Autodesk Fusion 360 part; units mm, degrees
(part 2 of 2)
  line L91 (21.2817, 6.4213) -> (21.3731, 6.0822)
  line L92 (21.3731, 6.0822) -> (22.0486, 6.2643)
  line L93 (22.0486, 6.2643) -> (22.45, 5.8793)
  line L94 (22.45, 5.8793) -> (21.497, 5.6224)
  line L95 (21.497, 5.6224) -> (21.6223, 5.1575)
  line L96 (21.6223, 5.1575) -> (21.2627, 5.0606)
  line L97 (21.2627, 5.0606) -> (21.1374, 5.5255)
  line L98 (21.1374, 5.5255) -> (19.5423, 5.0955)
  spline S235 degree 2 poles (19.5423, 5.0955) (19.3445, 5.0422) (19.2946, 5.0026) knots 0 0 0 1 1 1
  spline S236 degree 2 poles (19.2946, 5.0026) (19.2446, 4.9629) (19.2261, 4.8987) knots 0 0 0 1 1 1
  spline S237 degree 2 poles (19.2261, 4.8987) (19.2076, 4.8345) (19.2353, 4.7317) knots 0 0 0 1 1 1
  spline S238 degree 2 poles (19.2353, 4.7317) (19.2561, 4.6547) (19.308, 4.5337) knots 0 0 0 1 1 1
  line L99 (19.0191, 3.968) -> (22.8775, 4.536)
  line L100 (22.8775, 4.536) -> (22.9473, 4.0623)
  line L101 (22.9473, 4.0623) -> (21.5629, 3.8585)
  spline S239 degree 2 poles (21.5629, 3.8585) (21.996, 3.5834) (22.0703, 3.0781) knots 0 0 0 1 1 1
  spline S240 degree 2 poles (22.0703, 3.0781) (22.1161, 2.7675) (22.0274, 2.5205) knots 0 0 0 1 1 1
  spline S241 degree 2 poles (22.0274, 2.5205) (21.9387, 2.2735) (21.7374, 2.1431) knots 0 0 0 1 1 1
  spline S242 degree 2 poles (21.7374, 2.1431) (21.5361, 2.0126) (21.1255, 1.9522) knots 0 0 0 1 1 1
  line L102 (21.1255, 1.9522) -> (19.3542, 1.6914)
  line L103 (19.3542, 1.6914) -> (19.2845, 2.1652)
  line L104 (19.2845, 2.1652) -> (21.0558, 2.4259)
  spline S243 degree 2 poles (21.0558, 2.4259) (21.4111, 2.4782) (21.5503, 2.656) knots 0 0 0 1 1 1
  spline S244 degree 2 poles (21.5503, 2.656) (21.6895, 2.8338) (21.6481, 3.1154) knots 0 0 0 1 1 1
  spline S245 degree 2 poles (21.6481, 3.1154) (21.6171, 3.326) (21.4805, 3.4954) knots 0 0 0 1 1 1
  spline S246 degree 2 poles (21.4805, 3.4954) (21.344, 3.6649) (21.1455, 3.7164) knots 0 0 0 1 1 1
  spline S247 degree 2 poles (21.1455, 3.7164) (20.947, 3.7678) (20.618, 3.7194) knots 0 0 0 1 1 1
  line L105 (20.618, 3.7194) -> (19.0889, 3.4943)
  line L106 (19.0889, 3.4943) -> (19.0191, 3.968)
  line L107 (20.2952, -0.9828) -> (20.229, -1.477)
  spline S248 degree 2 poles (20.229, -1.477) (19.7966, -1.3556) (19.5604, -1.0366) knots 0 0 0 1 1 1
  spline S249 degree 2 poles (19.5604, -1.0366) (19.3241, -0.7176) (19.3291, -0.2255) knots 0 0 0 1 1 1
  spline S250 degree 2 poles (19.3291, -0.2255) (19.3353, 0.3943) (19.7207, 0.7536) knots 0 0 0 1 1 1
  spline S251 degree 2 poles (19.7207, 0.7536) (20.1061, 1.1129) (20.7951, 1.1059) knots 0 0 0 1 1 1
  spline S252 degree 2 poles (20.7951, 1.1059) (21.508, 1.0987) (21.898, 0.7277) knots 0 0 0 1 1 1
  spline S253 degree 2 poles (21.898, 0.7277) (22.288, 0.3566) (22.2821, -0.2286) knots 0 0 0 1 1 1
  spline S254 degree 2 poles (22.2821, -0.2286) (22.2764, -0.7953) (21.8871, -1.1505) knots 0 0 0 1 1 1
  spline S255 degree 2 poles (21.8871, -1.1505) (21.4977, -1.5057) (20.7981, -1.4987) knots 0 0 0 1 1 1
  spline S256 degree 2 poles (20.7981, -1.4987) (20.7556, -1.4982) (20.6705, -1.4947) knots 0 0 0 1 1 1
  line L108 (20.6705, -1.4947) -> (20.6917, 0.6121)
  spline S257 degree 2 poles (20.6917, 0.6121) (20.2259, 0.5902) (19.9761, 0.356) knots 0 0 0 1 1 1
  spline S258 degree 2 poles (19.9761, 0.356) (19.7263, 0.1217) (19.7228, -0.2321) knots 0 0 0 1 1 1
  spline S259 degree 2 poles (19.7228, -0.2321) (19.7201, -0.4955) (19.8566, -0.6831) knots 0 0 0 1 1 1
  spline S260 degree 2 poles (19.8566, -0.6831) (19.993, -0.8707) (20.2952, -0.9828) knots 0 0 0 1 1 1
  line L109 (21.0851, 0.5816) -> (21.0692, -0.9959)
  spline S261 degree 2 poles (21.0692, -0.9959) (21.426, -0.9676) (21.6057, -0.8204) knots 0 0 0 1 1 1
  spline S262 degree 2 poles (21.6057, -0.8204) (21.8847, -0.5944) (21.8884, -0.23) knots 0 0 0 1 1 1
  spline S263 degree 2 poles (21.8884, -0.23) (21.8917, 0.0999) (21.6732, 0.3269) knots 0 0 0 1 1 1
  spline S264 degree 2 poles (21.6732, 0.3269) (21.4547, 0.5539) (21.0851, 0.5816) knots 0 0 0 1 1 1
  line L110 (19.1426, -3.6298) -> (22.8872, -4.7198)
  line L111 (22.8872, -4.7198) -> (22.6701, -5.4656)
  line L112 (22.6701, -5.4656) -> (19.7607, -5.5802)
  spline S265 degree 2 poles (19.7607, -5.5802) (19.3547, -5.595) (19.1544, -5.5977) knots 0 0 0 1 1 1
  spline S266 degree 2 poles (19.1544, -5.5977) (19.3401, -5.721) (19.6967, -5.9716) knots 0 0 0 1 1 1
  line L113 (19.6967, -5.9716) -> (22.0411, -7.6266)
  line L114 (22.0411, -7.6266) -> (21.847, -8.2932)
  line L115 (21.847, -8.2932) -> (18.1024, -7.2032)
  line L116 (18.1024, -7.2032) -> (18.2415, -6.7256)
  line L117 (18.2415, -6.7256) -> (21.3756, -7.6379)
  line L118 (21.3756, -7.6379) -> (18.5582, -5.6375)
  line L119 (18.5582, -5.6375) -> (18.6883, -5.1905)
  line L120 (18.6883, -5.1905) -> (22.1913, -5.0353)
  line L121 (22.1913, -5.0353) -> (19.0035, -4.1074)
  line L122 (19.0035, -4.1074) -> (19.1426, -3.6298)
  line L123 (18.9246, -8.4047) -> (18.7313, -8.8535)
  spline S267 degree 2 poles (18.7313, -8.8535) (18.4572, -8.7452) (18.2322, -8.7675) knots 0 0 0 1 1 1
  spline S268 degree 2 poles (18.2322, -8.7675) (18.0072, -8.7899) (17.7791, -8.9692) knots 0 0 0 1 1 1
  spline S269 degree 2 poles (17.7791, -8.9692) (17.5511, -9.1486) (17.3935, -9.4414) knots 0 0 0 1 1 1
  spline S270 degree 2 poles (17.3935, -9.4414) (17.2535, -9.7014) (17.2236, -9.9421) knots 0 0 0 1 1 1
  spline S271 degree 2 poles (17.2236, -9.9421) (17.1936, -10.1828) (17.276, -10.3526) knots 0 0 0 1 1 1
  spline S272 degree 2 poles (17.276, -10.3526) (17.3583, -10.5223) (17.5176, -10.6081) knots 0 0 0 1 1 1
  spline S273 degree 2 poles (17.5176, -10.6081) (17.6792, -10.6951) (17.8503, -10.6663) knots 0 0 0 1 1 1
  spline S274 degree 2 poles (17.8503, -10.6663) (18.0214, -10.6376) (18.2194, -10.4663) knots 0 0 0 1 1 1
  spline S275 degree 2 poles (18.2194, -10.4663) (18.3477, -10.3571) (18.7161, -9.9451) knots 0 0 0 1 1 1
  spline S276 degree 2 poles (18.7161, -9.9451) (19.0844, -9.5331) (19.2873, -9.3976) knots 0 0 0 1 1 1
  spline S277 degree 2 poles (19.2873, -9.3976) (19.5486, -9.2211) (19.8044, -9.2032) knots 0 0 0 1 1 1
  spline S278 degree 2 poles (19.8044, -9.2032) (20.0603, -9.1854) (20.2969, -9.3128) knots 0 0 0 1 1 1
  spline S279 degree 2 poles (20.2969, -9.3128) (20.5569, -9.4528) (20.7034, -9.722) knots 0 0 0 1 1 1
  spline S280 degree 2 poles (20.7034, -9.722) (20.85, -9.9913) (20.8145, -10.3378) knots 0 0 0 1 1 1
  spline S281 degree 2 poles (20.8145, -10.3378) (20.779, -10.6843) (20.5923, -11.031) knots 0 0 0 1 1 1
  spline S282 degree 2 poles (20.5923, -11.031) (20.3868, -11.4127) (20.1068, -11.6382) knots 0 0 0 1 1 1
  spline S283 degree 2 poles (20.1068, -11.6382) (19.8268, -11.8636) (19.5033, -11.8918) knots 0 0 0 1 1 1
  spline S284 degree 2 poles (19.5033, -11.8918) (19.1799, -11.9201) (18.8715, -11.7691) knots 0 0 0 1 1 1
  line L124 (18.8715, -11.7691) -> (19.0733, -11.3158)
  spline S285 degree 2 poles (19.0733, -11.3158) (19.4178, -11.456) (19.6932, -11.3429) knots 0 0 0 1 1 1
  spline S286 degree 2 poles (19.6932, -11.3429) (19.9686, -11.2299) (20.1817, -10.834) knots 0 0 0 1 1 1
  spline S287 degree 2 poles (20.1817, -10.834) (20.4037, -10.4218) (20.3542, -10.1519) knots 0 0 0 1 1 1
  spline S288 degree 2 poles (20.3542, -10.1519) (20.3046, -9.882) (20.0915, -9.7672) knots 0 0 0 1 1 1
  spline S289 degree 2 poles (20.0915, -9.7672) (19.9064, -9.6675) (19.7151, -9.7367) knots 0 0 0 1 1 1
  spline S290 degree 2 poles (19.7151, -9.7367) (19.525, -9.8036) (19.1014, -10.2901) knots 0 0 0 1 1 1
  spline S291 degree 2 poles (19.1014, -10.2901) (18.6778, -10.7765) (18.4731, -10.9322) knots 0 0 0 1 1 1
  spline S292 degree 2 poles (18.4731, -10.9322) (18.1735, -11.1576) (17.8845, -11.1863) knots 0 0 0 1 1 1
  spline S293 degree 2 poles (17.8845, -11.1863) (17.5956, -11.2151) (17.3192, -11.0662) knots 0 0 0 1 1 1
  spline S294 degree 2 poles (17.3192, -11.0662) (17.0452, -10.9187) (16.8873, -10.6312) knots 0 0 0 1 1 1
  spline S295 degree 2 poles (16.8873, -10.6312) (16.7293, -10.3437) (16.7529, -9.9772) knots 0 0 0 1 1 1
  spline S296 degree 2 poles (16.7529, -9.9772) (16.7765, -9.6108) (16.9746, -9.243) knots 0 0 0 1 1 1
  spline S297 degree 2 poles (16.9746, -9.243) (17.2255, -8.7769) (17.531, -8.535) knots 0 0 0 1 1 1
  spline S298 degree 2 poles (17.531, -8.535) (17.8365, -8.2931) (18.2059, -8.2609) knots 0 0 0 1 1 1
  spline S299 degree 2 poles (18.2059, -8.2609) (18.5753, -8.2286) (18.9246, -8.4047) knots 0 0 0 1 1 1
  line L125 (15.066, -12.3544) -> (17.8311, -15.1046)
  line L126 (17.8311, -15.1046) -> (17.2833, -15.6554)
  line L127 (17.2833, -15.6554) -> (14.6745, -14.3626)
  spline S300 degree 2 poles (14.6745, -14.3626) (14.3109, -14.1811) (14.1339, -14.0875) knots 0 0 0 1 1 1
  spline S301 degree 2 poles (14.1339, -14.0875) (14.2379, -14.2848) (14.4308, -14.6755) knots 0 0 0 1 1 1
  line L128 (14.4308, -14.6755) -> (15.6962, -17.2511)
  line L129 (15.6962, -17.2511) -> (15.2066, -17.7434)
  line L130 (15.2066, -17.7434) -> (12.4414, -14.9932)
  line L131 (12.4414, -14.9932) -> (12.7922, -14.6405)
  line L132 (12.7922, -14.6405) -> (15.1066, -16.9423)
  line L133 (15.1066, -16.9423) -> (13.5914, -13.8369)
  line L134 (13.5914, -13.8369) -> (13.9197, -13.5068)
  line L135 (13.9197, -13.5068) -> (17.0691, -15.0484)
  line L136 (17.0691, -15.0484) -> (14.7152, -12.7071)
  line L137 (14.7152, -12.7071) -> (15.066, -12.3544)
  line L138 (11.1944, -14.5207) -> (11.4925, -14.8614)
  spline S302 degree 2 poles (11.4925, -14.8614) (11.3389, -14.9151) (11.2424, -14.9813) knots 0 0 0 1 1 1
  spline S303 degree 2 poles (11.2424, -14.9813) (11.1107, -15.0715) (11.0618, -15.1695) knots 0 0 0 1 1 1
  spline S304 degree 2 poles (11.0618, -15.1695) (11.0129, -15.2676) (11.0166, -15.3811) knots 0 0 0 1 1 1
  spline S305 degree 2 poles (11.0166, -15.3811) (11.0199, -15.466) (11.0974, -15.7579) knots 0 0 0 1 1 1
  spline S306 degree 2 poles (11.0974, -15.7579) (11.109, -15.7983) (11.1285, -15.8785) knots 0 0 0 1 1 1
  line L139 (11.1285, -15.8785) -> (13.6131, -17.6072)
  line L140 (13.6131, -17.6072) -> (13.1874, -17.899)
  line L141 (13.1874, -17.899) -> (11.7775, -16.8818)
  spline S307 degree 2 poles (11.7775, -16.8818) (11.5071, -16.6898) (11.2385, -16.4578) knots 0 0 0 1 1 1
  spline S308 degree 2 poles (11.2385, -16.4578) (11.357, -16.7766) (11.4401, -17.1002) knots 0 0 0 1 1 1
  line L142 (11.4401, -17.1002) -> (11.873, -18.7999)
  line L143 (11.873, -18.7999) -> (11.478, -19.0706)
  line L144 (11.478, -19.0706) -> (10.7402, -16.0931)
  spline S309 degree 2 poles (10.7402, -16.0931) (10.6196, -15.6113) (10.5993, -15.4123) knots 0 0 0 1 1 1
  spline S310 degree 2 poles (10.5993, -15.4123) (10.5708, -15.1449) (10.6444, -14.9605) knots 0 0 0 1 1 1
  spline S311 degree 2 poles (10.6444, -14.9605) (10.718, -14.7762) (10.9068, -14.6469) knots 0 0 0 1 1 1
  spline S312 degree 2 poles (10.9068, -14.6469) (11.0209, -14.5687) (11.1944, -14.5207) knots 0 0 0 1 1 1
  line L145 (10.0619, -17.5995) -> (9.6708, -17.8766)
  spline S313 degree 2 poles (9.6708, -17.8766) (9.5086, -17.6394) (9.2779, -17.5845) knots 0 0 0 1 1 1
  spline S314 degree 2 poles (9.2779, -17.5845) (9.0473, -17.5296) (8.7542, -17.675) knots 0 0 0 1 1 1
  spline S315 degree 2 poles (8.7542, -17.675) (8.4586, -17.8216) (8.3753, -18.0128) knots 0 0 0 1 1 1
  spline S316 degree 2 poles (8.3753, -18.0128) (8.292, -18.2041) (8.3724, -18.3662) knots 0 0 0 1 1 1
  spline S317 degree 2 poles (8.3724, -18.3662) (8.4445, -18.5116) (8.6122, -18.5323) knots 0 0 0 1 1 1
  spline S318 degree 2 poles (8.6122, -18.5323) (8.7287, -18.5458) (9.1228, -18.4602) knots 0 0 0 1 1 1
  spline S319 degree 2 poles (9.1228, -18.4602) (9.6538, -18.3453) (9.8793, -18.3419) knots 0 0 0 1 1 1
  spline S320 degree 2 poles (9.8793, -18.3419) (10.1047, -18.3385) (10.2751, -18.4455) knots 0 0 0 1 1 1
  spline S321 degree 2 poles (10.2751, -18.4455) (10.4455, -18.5525) (10.5377, -18.7384) knots 0 0 0 1 1 1
  spline S322 degree 2 poles (10.5377, -18.7384) (10.6216, -18.9077) (10.6157, -19.0903) knots 0 0 0 1 1 1
  spline S323 degree 2 poles (10.6157, -19.0903) (10.6097, -19.2729) (10.5235, -19.4344) knots 0 0 0 1 1 1
  spline S324 degree 2 poles (10.5235, -19.4344) (10.4601, -19.5579) (10.3127, -19.6948) knots 0 0 0 1 1 1
  spline S325 degree 2 poles (10.3127, -19.6948) (10.1653, -19.8318) (9.9675, -19.9299) knots 0 0 0 1 1 1
  spline S326 degree 2 poles (9.9675, -19.9299) (9.6696, -20.0776) (9.4018, -20.1035) knots 0 0 0 1 1 1
  spline S327 degree 2 poles (9.4018, -20.1035) (9.1341, -20.1294) (8.9541, -20.0361) knots 0 0 0 1 1 1
  spline S328 degree 2 poles (8.9541, -20.0361) (8.7742, -19.9427) (8.6119, -19.7173) knots 0 0 0 1 1 1
  line L146 (8.6119, -19.7173) -> (9.003, -19.4521)
  spline S329 degree 2 poles (9.003, -19.4521) (9.1285, -19.6333) (9.3199, -19.675) knots 0 0 0 1 1 1
  spline S330 degree 2 poles (9.3199, -19.675) (9.5113, -19.7166) (9.7616, -19.5925) knots 0 0 0 1 1 1
  spline S331 degree 2 poles (9.7616, -19.5925) (10.0571, -19.446) (10.135, -19.2856) knots 0 0 0 1 1 1
  spline S332 degree 2 poles (10.135, -19.2856) (10.2128, -19.1252) (10.1478, -18.9942) knots 0 0 0 1 1 1
  spline S333 degree 2 poles (10.1478, -18.9942) (10.1064, -18.9107) (10.0209, -18.87) knots 0 0 0 1 1 1
  spline S334 degree 2 poles (10.0209, -18.87) (9.9342, -18.8269) (9.7997, -18.8372) knots 0 0 0 1 1 1
  spline S335 degree 2 poles (9.7997, -18.8372) (9.7236, -18.8453) (9.3664, -18.9155) knots 0 0 0 1 1 1
  spline S336 degree 2 poles (9.3664, -18.9155) (8.8509, -19.0197) (8.6326, -19.0315) knots 0 0 0 1 1 1
  spline S337 degree 2 poles (8.6326, -19.0315) (8.4142, -19.0433) (8.2385, -18.9463) knots 0 0 0 1 1 1
  spline S338 degree 2 poles (8.2385, -18.9463) (8.0627, -18.8494) (7.9539, -18.6301) knots 0 0 0 1 1 1
  spline S339 degree 2 poles (7.9539, -18.6301) (7.8476, -18.4156) (7.8787, -18.1641) knots 0 0 0 1 1 1
  spline S340 degree 2 poles (7.8787, -18.1641) (7.9099, -17.9126) (8.0944, -17.6919) knots 0 0 0 1 1 1
  spline S341 degree 2 poles (8.0944, -17.6919) (8.2789, -17.4712) (8.5768, -17.3234) knots 0 0 0 1 1 1
  spline S342 degree 2 poles (8.5768, -17.3234) (9.0702, -17.0788) (9.4304, -17.1555) knots 0 0 0 1 1 1
  spline S343 degree 2 poles (9.4304, -17.1555) (9.7907, -17.2322) (10.0619, -17.5995) knots 0 0 0 1 1 1
  line L147 (6.2103, -18.8357) -> (5.9999, -18.4623)
  spline S344 degree 2 poles (5.9999, -18.4623) (6.1751, -18.3528) (6.3249, -18.2979) knots 0 0 0 1 1 1
  spline S345 degree 2 poles (6.3249, -18.2979) (6.5697, -18.2082) (6.733, -18.2363) knots 0 0 0 1 1 1
  spline S346 degree 2 poles (6.733, -18.2363) (6.8963, -18.2643) (6.9974, -18.3703) knots 0 0 0 1 1 1
  spline S347 degree 2 poles (6.9974, -18.3703) (7.0986, -18.4763) (7.2468, -18.881) knots 0 0 0 1 1 1
  line L148 (7.2468, -18.881) -> (7.806, -20.4072)
  line L149 (7.806, -20.4072) -> (8.1357, -20.2865)
  line L150 (8.1357, -20.2865) -> (8.2638, -20.6362)
  line L151 (8.2638, -20.6362) -> (7.9341, -20.757)
  line L152 (7.9341, -20.757) -> (8.1747, -21.4139)
  line L153 (8.1747, -21.4139) -> (7.8264, -21.8475)
  line L154 (7.8264, -21.8475) -> (7.4869, -20.9208)
  line L155 (7.4869, -20.9208) -> (7.0348, -21.0864)
  line L156 (7.0348, -21.0864) -> (6.9067, -20.7367)
  line L157 (6.9067, -20.7367) -> (7.3588, -20.571)
  line L158 (7.3588, -20.571) -> (6.7905, -19.0198)
  spline S348 degree 2 poles (6.7905, -19.0198) (6.7201, -18.8275) (6.6762, -18.7812) knots 0 0 0 1 1 1
  spline S349 degree 2 poles (6.6762, -18.7812) (6.6324, -18.7349) (6.5668, -18.7221) knots 0 0 0 1 1 1
  spline S350 degree 2 poles (6.5668, -18.7221) (6.5012, -18.7094) (6.4012, -18.746) knots 0 0 0 1 1 1
  spline S351 degree 2 poles (6.4012, -18.746) (6.3263, -18.7734) (6.2103, -18.8357) knots 0 0 0 1 1 1
  line L159 (6.5393, -21.7845) -> (6.692, -22.3136)
  line L160 (6.692, -22.3136) -> (6.2319, -22.4464)
  line L161 (6.2319, -22.4464) -> (6.0792, -21.9173)
  line L162 (6.0792, -21.9173) -> (6.5393, -21.7845)
  line L163 (5.6108, -18.5665) -> (6.394, -21.281)
  line L164 (6.394, -21.281) -> (5.9339, -21.4137)
  line L165 (5.9339, -21.4137) -> (5.1507, -18.6993)
  line L166 (5.1507, -18.6993) -> (5.6108, -18.5665)
  line L167 (2.4912, -18.1527) -> (2.7274, -19.5158)
  spline S352 degree 2 poles (2.7274, -19.5158) (2.8107, -19.342) (2.9908, -19.2055) knots 0 0 0 1 1 1
  spline S353 degree 2 poles (2.9908, -19.2055) (3.171, -19.069) (3.3938, -19.0304) knots 0 0 0 1 1 1
  spline S354 degree 2 poles (3.3938, -19.0304) (3.8893, -18.9445) (4.3156, -19.2783) knots 0 0 0 1 1 1
  spline S355 degree 2 poles (4.3156, -19.2783) (4.742, -19.6121) (4.8615, -20.3015) knots 0 0 0 1 1 1
  spline S356 degree 2 poles (4.8615, -20.3015) (4.9342, -20.7209) (4.8464, -21.079) knots 0 0 0 1 1 1
  spline S357 degree 2 poles (4.8464, -21.079) (4.7586, -21.4371) (4.5118, -21.6567) knots 0 0 0 1 1 1
  spline S358 degree 2 poles (4.5118, -21.6567) (4.265, -21.8763) (3.9348, -21.9336) knots 0 0 0 1 1 1
  spline S359 degree 2 poles (3.9348, -21.9336) (3.4184, -22.0231) (3.0468, -21.6393) knots 0 0 0 1 1 1
  line L168 (3.0468, -21.6393) -> (3.1113, -22.0115)
  line L169 (3.1113, -22.0115) -> (2.6866, -22.0851)
  line L170 (2.6866, -22.0851) -> (2.0193, -18.2345)
  line L171 (2.0193, -18.2345) -> (2.4912, -18.1527)
  spline S360 degree 2 poles (4.3734, -20.3672) (4.2803, -19.8298) (4.0083, -19.6002) knots 0 0 0 1 1 1
  spline S361 degree 2 poles (4.0083, -19.6002) (3.7363, -19.3706) (3.4218, -19.4251) knots 0 0 0 1 1 1
  spline S362 degree 2 poles (3.4218, -19.4251) (3.1203, -19.4774) (2.947, -19.7706) knots 0 0 0 1 1 1
  spline S363 degree 2 poles (2.947, -19.7706) (2.7738, -20.0639) (2.8642, -20.5855) knots 0 0 0 1 1 1
  spline S364 degree 2 poles (2.8642, -20.5855) (2.9605, -21.1412) (3.2384, -21.3819) knots 0 0 0 1 1 1
  spline S365 degree 2 poles (3.2384, -21.3819) (3.5164, -21.6227) (3.8257, -21.5691) knots 0 0 0 1 1 1
  spline S366 degree 2 poles (3.8257, -21.5691) (4.1324, -21.5159) (4.3008, -21.2181) knots 0 0 0 1 1 1
  spline S367 degree 2 poles (4.3008, -21.2181) (4.4692, -20.9203) (4.3734, -20.3672) knots 0 0 0 1 1 1
  line L172 (-0.3977, -19.4026) -> (-0.3913, -19.8176)
  spline S368 degree 2 poles (-0.3913, -19.8176) (-0.0688, -19.3337) (0.4978, -19.325) knots 0 0 0 1 1 1
  spline S369 degree 2 poles (0.4978, -19.325) (0.7478, -19.3212) (0.966, -19.4136) knots 0 0 0 1 1 1
  spline S370 degree 2 poles (0.966, -19.4136) (1.1843, -19.506) (1.2916, -19.6494) knots 0 0 0 1 1 1
  spline S371 degree 2 poles (1.2916, -19.6494) (1.3989, -19.7927) (1.4447, -20.0022) knots 0 0 0 1 1 1
  spline S372 degree 2 poles (1.4447, -20.0022) (1.4761, -20.1428) (1.4808, -20.4487) knots 0 0 0 1 1 1
  line L173 (1.4808, -20.4487) -> (1.5077, -22.1989)
  line L174 (1.5077, -22.1989) -> (1.0289, -22.2063)
  line L175 (1.0289, -22.2063) -> (1.0048, -20.6396)
  spline S373 degree 2 poles (1.0048, -20.6396) (0.9991, -20.2645) (0.9678, -20.1346) knots 0 0 0 1 1 1
  spline S374 degree 2 poles (0.9678, -20.1346) (0.9197, -19.9464) (0.7717, -19.841) knots 0 0 0 1 1 1
  spline S375 degree 2 poles (0.7717, -19.841) (0.6238, -19.7355) (0.4083, -19.7388) knots 0 0 0 1 1 1
  spline S376 degree 2 poles (0.4083, -19.7388) (0.1929, -19.7421) (0.0057, -19.8554) knots 0 0 0 1 1 1
  spline S377 degree 2 poles (0.0057, -19.8554) (-0.1815, -19.9687) (-0.257, -20.1601) knots 0 0 0 1 1 1
  spline S378 degree 2 poles (-0.257, -20.1601) (-0.3326, -20.3515) (-0.327, -20.7132) knots 0 0 0 1 1 1
  line L176 (-0.327, -20.7132) -> (-0.3037, -22.2268)
  line L177 (-0.3037, -22.2268) -> (-0.7825, -22.2341)
  line L178 (-0.7825, -22.2341) -> (-0.8259, -19.4092)
  line L179 (-0.8259, -19.4092) -> (-0.3977, -19.4026)
  line L180 (-3.6213, -19.9937) -> (-4.1026, -19.8636)
  spline S379 degree 2 poles (-4.1026, -19.8636) (-3.9259, -19.4507) (-3.5788, -19.2581) knots 0 0 0 1 1 1
  spline S380 degree 2 poles (-3.5788, -19.2581) (-3.2317, -19.0655) (-2.7445, -19.1346) knots 0 0 0 1 1 1
  spline S381 degree 2 poles (-2.7445, -19.1346) (-2.1308, -19.2216) (-1.8248, -19.6506) knots 0 0 0 1 1 1
  spline S382 degree 2 poles (-1.8248, -19.6506) (-1.5189, -20.0795) (-1.6156, -20.7617) knots 0 0 0 1 1 1
  spline S383 degree 2 poles (-1.6156, -20.7617) (-1.7157, -21.4676) (-2.1345, -21.8059) knots 0 0 0 1 1 1
  spline S384 degree 2 poles (-2.1345, -21.8059) (-2.5533, -22.1442) (-3.1327, -22.062) knots 0 0 0 1 1 1
  spline S385 degree 2 poles (-3.1327, -22.062) (-3.6938, -21.9824) (-3.9952, -21.5501) knots 0 0 0 1 1 1
  spline S386 degree 2 poles (-3.9952, -21.5501) (-4.2966, -21.1177) (-4.1984, -20.425) knots 0 0 0 1 1 1
  spline S387 degree 2 poles (-4.1984, -20.425) (-4.1924, -20.3829) (-4.1778, -20.299) knots 0 0 0 1 1 1
  line L181 (-4.1778, -20.299) -> (-2.0917, -20.5948)
  spline S388 degree 2 poles (-2.0917, -20.5948) (-2.0527, -20.1301) (-2.2524, -19.8519) knots 0 0 0 1 1 1
  spline S389 degree 2 poles (-2.2524, -19.8519) (-2.4521, -19.5737) (-2.8024, -19.524) knots 0 0 0 1 1 1
  spline S390 degree 2 poles (-2.8024, -19.524) (-3.0631, -19.4871) (-3.2669, -19.5979) knots 0 0 0 1 1 1
  spline S391 degree 2 poles (-3.2669, -19.5979) (-3.4707, -19.7087) (-3.6213, -19.9937) knots 0 0 0 1 1 1
  line L182 (-2.1734, -20.9809) -> (-3.7353, -20.7594)
  spline S392 degree 2 poles (-3.7353, -20.7594) (-3.7537, -21.1168) (-3.6313, -21.3142) knots 0 0 0 1 1 1
  spline S393 degree 2 poles (-3.6313, -21.3142) (-3.4436, -21.6203) (-3.0827, -21.6714) knots 0 0 0 1 1 1
  spline S394 degree 2 poles (-3.0827, -21.6714) (-2.7561, -21.7178) (-2.5026, -21.5307) knots 0 0 0 1 1 1
  spline S395 degree 2 poles (-2.5026, -21.5307) (-2.249, -21.3436) (-2.1734, -20.9809) knots 0 0 0 1 1 1
  spline S396 degree 2 poles (-6.3827, -19.8486) (-6.6703, -20.5788) (-7.2147, -20.7704) knots 0 0 0 1 1 1
  spline S397 degree 2 poles (-7.2147, -20.7704) (-7.6688, -20.9289) (-8.1564, -20.7369) knots 0 0 0 1 1 1
  spline S398 degree 2 poles (-8.1564, -20.7369) (-8.6985, -20.5234) (-8.9027, -20.0327) knots 0 0 0 1 1 1
  spline S399 degree 2 poles (-8.9027, -20.0327) (-9.1069, -19.542) (-8.8603, -18.9158) knots 0 0 0 1 1 1
  spline S400 degree 2 poles (-8.8603, -18.9158) (-8.6604, -18.4083) (-8.3937, -18.1774) knots 0 0 0 1 1 1
  spline S401 degree 2 poles (-8.3937, -18.1774) (-8.1269, -17.9466) (-7.7727, -17.9002) knots 0 0 0 1 1 1
  spline S402 degree 2 poles (-7.7727, -17.9002) (-7.4185, -17.8538) (-7.0744, -17.9893) knots 0 0 0 1 1 1
  spline S403 degree 2 poles (-7.0744, -17.9893) (-6.5224, -18.2067) (-6.3215, -18.6947) knots 0 0 0 1 1 1
  spline S404 degree 2 poles (-6.3215, -18.6947) (-6.1205, -19.1827) (-6.3827, -19.8486) knots 0 0 0 1 1 1
  spline S405 degree 2 poles (-6.8407, -19.6682) (-6.6418, -19.1633) (-6.7632, -18.8253) knots 0 0 0 1 1 1
  spline S406 degree 2 poles (-6.7632, -18.8253) (-6.8845, -18.4873) (-7.2187, -18.3557) knots 0 0 0 1 1 1
  spline S407 degree 2 poles (-7.2187, -18.3557) (-7.5504, -18.2251) (-7.8701, -18.3908) knots 0 0 0 1 1 1
  spline S408 degree 2 poles (-7.8701, -18.3908) (-8.1898, -18.5565) (-8.3936, -19.0738) knots 0 0 0 1 1 1
  spline S409 degree 2 poles (-8.3936, -19.0738) (-8.5856, -19.5615) (-8.463, -19.8999) knots 0 0 0 1 1 1
  spline S410 degree 2 poles (-8.463, -19.8999) (-8.3404, -20.2384) (-8.0112, -20.3681) knots 0 0 0 1 1 1
  spline S411 degree 2 poles (-8.0112, -20.3681) (-7.677, -20.4997) (-7.3583, -20.3364) knots 0 0 0 1 1 1
  spline S412 degree 2 poles (-7.3583, -20.3364) (-7.0395, -20.1732) (-6.8407, -19.6682) knots 0 0 0 1 1 1
  line L183 (-8.9179, -17.2264) -> (-10.0878, -19.3823)
  line L184 (-10.0878, -19.3823) -> (-9.716, -19.584)
  line L185 (-9.716, -19.584) -> (-9.8936, -19.9114)
  line L186 (-9.8936, -19.9114) -> (-10.2654, -19.7096)
  line L187 (-10.2654, -19.7096) -> (-10.4088, -19.9738)
  spline S413 degree 2 poles (-10.4088, -19.9738) (-10.5445, -20.224) (-10.6549, -20.3215) knots 0 0 0 1 1 1
  spline S414 degree 2 poles (-10.6549, -20.3215) (-10.8045, -20.4522) (-11.0129, -20.4708) knots 0 0 0 1 1 1
  spline S415 degree 2 poles (-11.0129, -20.4708) (-11.2212, -20.4894) (-11.4972, -20.3397) knots 0 0 0 1 1 1
  spline S416 degree 2 poles (-11.4972, -20.3397) (-11.6749, -20.2433) (-11.8671, -20.0844) knots 0 0 0 1 1 1
  line L188 (-11.8671, -20.0844) -> (-11.6048, -19.7516)
  spline S417 degree 2 poles (-11.6048, -19.7516) (-11.4865, -19.846) (-11.3696, -19.9095) knots 0 0 0 1 1 1
  spline S418 degree 2 poles (-11.3696, -19.9095) (-11.1779, -20.0135) (-11.054, -19.9748) knots 0 0 0 1 1 1
  spline S419 degree 2 poles (-11.054, -19.9748) (-10.9301, -19.9361) (-10.8083, -19.7117) knots 0 0 0 1 1 1
  line L189 (-10.8083, -19.7117) -> (-10.6839, -19.4825)
  line L190 (-10.6839, -19.4825) -> (-11.168, -19.2199)
  line L191 (-11.168, -19.2199) -> (-10.9903, -18.8925)
  line L192 (-10.9903, -18.8925) -> (-10.5063, -19.1552)
  line L193 (-10.5063, -19.1552) -> (-9.3365, -16.9993)
  line L194 (-9.3365, -16.9993) -> (-8.9179, -17.2264)
  line L195 (-11.5378, -15.5911) -> (-13.899, -18.695)
  line L196 (-13.899, -18.695) -> (-14.2801, -18.4051)
  line L197 (-14.2801, -18.4051) -> (-11.9189, -15.3011)
  line L198 (-11.9189, -15.3011) -> (-11.5378, -15.5911)
  line L199 (-14.5469, -14.1862) -> (-14.8636, -13.801)
  spline S420 degree 2 poles (-14.8636, -13.801) (-14.4801, -13.5672) (-14.0856, -13.6116) knots 0 0 0 1 1 1
  spline S421 degree 2 poles (-14.0856, -13.6116) (-13.6912, -13.656) (-13.3344, -13.995) knots 0 0 0 1 1 1
  spline S422 degree 2 poles (-13.3344, -13.995) (-12.8849, -14.4219) (-12.8845, -14.9487) knots 0 0 0 1 1 1
  spline S423 degree 2 poles (-12.8845, -14.9487) (-12.8841, -15.4756) (-13.3586, -15.9752) knots 0 0 0 1 1 1
  spline S424 degree 2 poles (-13.3586, -15.9752) (-13.8496, -16.4921) (-14.387, -16.5248) knots 0 0 0 1 1 1
  spline S425 degree 2 poles (-14.387, -16.5248) (-14.9243, -16.5575) (-15.3487, -16.1544) knots 0 0 0 1 1 1
  spline S426 degree 2 poles (-15.3487, -16.1544) (-15.7595, -15.7642) (-15.7543, -15.2372) knots 0 0 0 1 1 1
  spline S427 degree 2 poles (-15.7543, -15.2372) (-15.749, -14.7101) (-15.2672, -14.2028) knots 0 0 0 1 1 1
  spline S428 degree 2 poles (-15.2672, -14.2028) (-15.2379, -14.172) (-15.1773, -14.1121) knots 0 0 0 1 1 1
  line L200 (-15.1773, -14.1121) -> (-13.6496, -15.5631)
  spline S429 degree 2 poles (-13.6496, -15.5631) (-13.3483, -15.2072) (-13.3496, -14.8647) knots 0 0 0 1 1 1
  spline S430 degree 2 poles (-13.3496, -14.8647) (-13.3509, -14.5223) (-13.6074, -14.2786) knots 0 0 0 1 1 1
  spline S431 degree 2 poles (-13.6074, -14.2786) (-13.7984, -14.0973) (-14.0287, -14.0693) knots 0 0 0 1 1 1
  spline S432 degree 2 poles (-14.0287, -14.0693) (-14.259, -14.0414) (-14.5469, -14.1862) knots 0 0 0 1 1 1
  line L201 (-13.9401, -15.8302) -> (-15.0839, -14.7438)
  spline S433 degree 2 poles (-15.0839, -14.7438) (-15.3063, -15.0243) (-15.321, -15.2561) knots 0 0 0 1 1 1
  spline S434 degree 2 poles (-15.321, -15.2561) (-15.3456, -15.6143) (-15.0814, -15.8653) knots 0 0 0 1 1 1
  spline S435 degree 2 poles (-15.0814, -15.8653) (-14.8422, -16.0924) (-14.5271, -16.0871) knots 0 0 0 1 1 1
  spline S436 degree 2 poles (-14.5271, -16.0871) (-14.2121, -16.0819) (-13.9401, -15.8302) knots 0 0 0 1 1 1
  line L202 (-15.8662, -11.1763) -> (-15.6239, -11.5486)
  line L203 (-15.6239, -11.5486) -> (-18.8928, -13.6757)
  line L204 (-18.8928, -13.6757) -> (-19.154, -13.2743)
  line L205 (-19.154, -13.2743) -> (-17.9878, -12.5155)
  spline S437 degree 2 poles (-17.9878, -12.5155) (-18.4721, -12.4688) (-18.7289, -12.0741) knots 0 0 0 1 1 1
  spline S438 degree 2 poles (-18.7289, -12.0741) (-18.8711, -11.8556) (-18.91, -11.6032) knots 0 0 0 1 1 1
  spline S439 degree 2 poles (-18.91, -11.6032) (-18.9488, -11.3507) (-18.8714, -11.121) knots 0 0 0 1 1 1
  spline S440 degree 2 poles (-18.8714, -11.121) (-18.7939, -10.8913) (-18.6151, -10.6734) knots 0 0 0 1 1 1
  spline S441 degree 2 poles (-18.6151, -10.6734) (-18.4364, -10.4555) (-18.1799, -10.2886) knots 0 0 0 1 1 1
  spline S442 degree 2 poles (-18.1799, -10.2886) (-17.5712, -9.8925) (-17.0431, -9.9774) knots 0 0 0 1 1 1
  spline S443 degree 2 poles (-17.0431, -9.9774) (-16.515, -10.0622) (-16.2407, -10.4836) knots 0 0 0 1 1 1
  spline S444 degree 2 poles (-16.2407, -10.4836) (-15.968, -10.9029) (-16.1628, -11.3692) knots 0 0 0 1 1 1
  line L206 (-16.1628, -11.3692) -> (-15.8662, -11.1763)
  spline S445 degree 2 poles (-17.0652, -11.9628) (-16.6393, -11.6856) (-16.5252, -11.4464) knots 0 0 0 1 1 1
  spline S446 degree 2 poles (-16.5252, -11.4464) (-16.3386, -11.0552) (-16.549, -10.7318) knots 0 0 0 1 1 1
  spline S447 degree 2 poles (-16.549, -10.7318) (-16.7202, -10.4687) (-17.0735, -10.4257) knots 0 0 0 1 1 1
  spline S448 degree 2 poles (-17.0735, -10.4257) (-17.4269, -10.3826) (-17.8795, -10.6772) knots 0 0 0 1 1 1
  spline S449 degree 2 poles (-17.8795, -10.6772) (-18.3433, -10.979) (-18.4444, -11.3066) knots 0 0 0 1 1 1
  spline S450 degree 2 poles (-18.4444, -11.3066) (-18.5454, -11.6342) (-18.3757, -11.895) knots 0 0 0 1 1 1
  spline S451 degree 2 poles (-18.3757, -11.895) (-18.2045, -12.1582) (-17.8511, -12.2012) knots 0 0 0 1 1 1
  spline S452 degree 2 poles (-17.8511, -12.2012) (-17.4978, -12.2442) (-17.0652, -11.9628) knots 0 0 0 1 1 1
  spline S453 degree 2 poles (-18.4484, -9.714) (-19.1648, -10.0344) (-19.6878, -9.7904) knots 0 0 0 1 1 1
  spline S454 degree 2 poles (-19.6878, -9.7904) (-20.1232, -9.5859) (-20.3371, -9.1075) knots 0 0 0 1 1 1
  spline S455 degree 2 poles (-20.3371, -9.1075) (-20.575, -8.5757) (-20.3776, -8.0823) knots 0 0 0 1 1 1
  spline S456 degree 2 poles (-20.3776, -8.0823) (-20.1801, -7.5888) (-19.5657, -7.314) knots 0 0 0 1 1 1
  spline S457 degree 2 poles (-19.5657, -7.314) (-19.0679, -7.0913) (-18.7157, -7.113) knots 0 0 0 1 1 1
  spline S458 degree 2 poles (-18.7157, -7.113) (-18.3636, -7.1347) (-18.0781, -7.3494) knots 0 0 0 1 1 1
  spline S459 degree 2 poles (-18.0781, -7.3494) (-17.7926, -7.5642) (-17.6416, -7.9017) knots 0 0 0 1 1 1
  spline S460 degree 2 poles (-17.6416, -7.9017) (-17.3994, -8.4433) (-17.5973, -8.9325) knots 0 0 0 1 1 1
  spline S461 degree 2 poles (-17.5973, -8.9325) (-17.7952, -9.4218) (-18.4484, -9.714) knots 0 0 0 1 1 1
  spline S462 degree 2 poles (-18.6494, -9.2647) (-18.154, -9.0431) (-18.0042, -8.7167) knots 0 0 0 1 1 1
  spline S463 degree 2 poles (-18.0042, -8.7167) (-17.8544, -8.3903) (-18.001, -8.0625) knots 0 0 0 1 1 1
  spline S464 degree 2 poles (-18.001, -8.0625) (-18.1466, -7.7371) (-18.491, -7.6318) knots 0 0 0 1 1 1
  spline S465 degree 2 poles (-18.491, -7.6318) (-18.8353, -7.5264) (-19.3429, -7.7535) knots 0 0 0 1 1 1
  spline S466 degree 2 poles (-19.3429, -7.7535) (-19.8213, -7.9675) (-19.9705, -8.2951) knots 0 0 0 1 1 1
  spline S467 degree 2 poles (-19.9705, -8.2951) (-20.1198, -8.6227) (-19.9753, -8.9456) knots 0 0 0 1 1 1
  spline S468 degree 2 poles (-19.9753, -8.9456) (-19.8287, -9.2735) (-19.4867, -9.3799) knots 0 0 0 1 1 1
  spline S469 degree 2 poles (-19.4867, -9.3799) (-19.1448, -9.4863) (-18.6494, -9.2647) knots 0 0 0 1 1 1
  spline S470 degree 2 poles (-19.2364, -4.4954) (-18.9486, -4.6931) (-18.7944, -4.9063) knots 0 0 0 1 1 1
  spline S471 degree 2 poles (-18.7944, -4.9063) (-18.6403, -5.1195) (-18.5666, -5.3917) knots 0 0 0 1 1 1
  spline S472 degree 2 poles (-18.5666, -5.3917) (-18.4449, -5.8411) (-18.5991, -6.1419) knots 0 0 0 1 1 1
  spline S473 degree 2 poles (-18.5991, -6.1419) (-18.7533, -6.4427) (-19.0949, -6.5351) knots 0 0 0 1 1 1
  spline S474 degree 2 poles (-19.0949, -6.5351) (-19.2951, -6.5894) (-19.4855, -6.5431) knots 0 0 0 1 1 1
  spline S475 degree 2 poles (-19.4855, -6.5431) (-19.6758, -6.4967) (-19.8159, -6.3762) knots 0 0 0 1 1 1
  spline S476 degree 2 poles (-19.8159, -6.3762) (-19.956, -6.2557) (-20.0574, -6.0847) knots 0 0 0 1 1 1
  spline S477 degree 2 poles (-20.0574, -6.0847) (-20.1302, -5.9583) (-20.238, -5.6926) knots 0 0 0 1 1 1
  spline S478 degree 2 poles (-20.238, -5.6926) (-20.4563, -5.1509) (-20.6203, -4.9114) knots 0 0 0 1 1 1
  spline S479 degree 2 poles (-20.6203, -4.9114) (-20.716, -4.9346) (-20.7417, -4.9415) knots 0 0 0 1 1 1
  spline S480 degree 2 poles (-20.7417, -4.9415) (-21.0242, -5.018) (-21.1043, -5.1802) knots 0 0 0 1 1 1
  spline S481 degree 2 poles (-21.1043, -5.1802) (-21.213, -5.3998) (-21.1184, -5.749) knots 0 0 0 1 1 1
  spline S482 degree 2 poles (-21.1184, -5.749) (-21.0301, -6.0752) (-20.8738, -6.1996) knots 0 0 0 1 1 1
  spline S483 degree 2 poles (-20.8738, -6.1996) (-20.7175, -6.324) (-20.4071, -6.3199) knots 0 0 0 1 1 1
  line L207 (-20.4071, -6.3199) -> (-20.3464, -6.7885)
  spline S484 degree 2 poles (-20.3464, -6.7885) (-20.6533, -6.8055) (-20.87, -6.7126) knots 0 0 0 1 1 1
  spline S485 degree 2 poles (-20.87, -6.7126) (-21.0867, -6.6196) (-21.2553, -6.3786) knots 0 0 0 1 1 1
  spline S486 degree 2 poles (-21.2553, -6.3786) (-21.4239, -6.1377) (-21.5191, -5.7859) knots 0 0 0 1 1 1
  spline S487 degree 2 poles (-21.5191, -5.7859) (-21.6136, -5.4366) (-21.5906, -5.1961) knots 0 0 0 1 1 1
  spline S488 degree 2 poles (-21.5906, -5.1961) (-21.5675, -4.9556) (-21.4707, -4.8192) knots 0 0 0 1 1 1
  spline S489 degree 2 poles (-21.4707, -4.8192) (-21.374, -4.6827) (-21.1951, -4.5902) knots 0 0 0 1 1 1
  spline S490 degree 2 poles (-21.1951, -4.5902) (-21.0833, -4.5351) (-20.7751, -4.4517) knots 0 0 0 1 1 1
  line L208 (-20.7751, -4.4517) -> (-20.1588, -4.2849)
  spline S491 degree 2 poles (-20.1588, -4.2849) (-19.5143, -4.1104) (-19.3515, -4.0346) knots 0 0 0 1 1 1
  spline S492 degree 2 poles (-19.3515, -4.0346) (-19.1888, -3.9588) (-19.0557, -3.8291) knots 0 0 0 1 1 1
  line L209 (-19.0557, -3.8291) -> (-18.9251, -4.3119)
  spline S493 degree 2 poles (-18.9251, -4.3119) (-19.0494, -4.4227) (-19.2364, -4.4954) knots 0 0 0 1 1 1
  spline S494 degree 2 poles (-20.2583, -4.8134) (-20.0874, -5.0372) (-19.8793, -5.5211) knots 0 0 0 1 1 1
  spline S495 degree 2 poles (-19.8793, -5.5211) (-19.761, -5.795) (-19.6777, -5.8992) knots 0 0 0 1 1 1
  spline S496 degree 2 poles (-19.6777, -5.8992) (-19.5943, -6.0034) (-19.4781, -6.0408) knots 0 0 0 1 1 1
  spline S497 degree 2 poles (-19.4781, -6.0408) (-19.3619, -6.0783) (-19.2412, -6.0456) knots 0 0 0 1 1 1
  spline S498 degree 2 poles (-19.2412, -6.0456) (-19.0563, -5.9955) (-18.9709, -5.8222) knots 0 0 0 1 1 1
  spline S499 degree 2 poles (-18.9709, -5.8222) (-18.8855, -5.6489) (-18.9585, -5.3793) knots 0 0 0 1 1 1
  spline S500 degree 2 poles (-18.9585, -5.3793) (-19.0308, -5.1122) (-19.204, -4.9359) knots 0 0 0 1 1 1
  spline S501 degree 2 poles (-19.204, -4.9359) (-19.3771, -4.7595) (-19.6064, -4.7168) knots 0 0 0 1 1 1
  spline S502 degree 2 poles (-19.6064, -4.7168) (-19.7832, -4.6848) (-20.0888, -4.7675) knots 0 0 0 1 1 1
  line L210 (-20.0888, -4.7675) -> (-20.2583, -4.8134)
  line L211 (-19.7031, -2.2675) -> (-19.2948, -2.137)
  spline S503 degree 2 poles (-19.2948, -2.137) (-19.223, -2.3308) (-19.1996, -2.4887) knots 0 0 0 1 1 1
  spline S504 degree 2 poles (-19.1996, -2.4887) (-19.1614, -2.7466) (-19.2219, -2.9008) knots 0 0 0 1 1 1
  spline S505 degree 2 poles (-19.2219, -2.9008) (-19.2824, -3.055) (-19.4067, -3.1326) knots 0 0 0 1 1 1
  spline S506 degree 2 poles (-19.4067, -3.1326) (-19.531, -3.2102) (-19.9573, -3.2734) knots 0 0 0 1 1 1
  line L212 (-19.9573, -3.2734) -> (-21.5651, -3.5119)
  line L213 (-21.5651, -3.5119) -> (-21.5136, -3.8592)
  line L214 (-21.5136, -3.8592) -> (-21.882, -3.9139)
  line L215 (-21.882, -3.9139) -> (-21.9336, -3.5665)
  line L216 (-21.9336, -3.5665) -> (-22.6256, -3.6692)
  line L217 (-22.6256, -3.6692) -> (-22.9797, -3.2403)
  line L218 (-22.9797, -3.2403) -> (-22.0034, -3.0955)
  line L219 (-22.0034, -3.0955) -> (-22.0741, -2.6192)
  line L220 (-22.0741, -2.6192) -> (-21.7057, -2.5645)
  line L221 (-21.7057, -2.5645) -> (-21.635, -3.0408)
  line L222 (-21.635, -3.0408) -> (-20.0008, -2.7985)
  spline S507 degree 2 poles (-20.0008, -2.7985) (-19.7982, -2.7684) (-19.744, -2.7348) knots 0 0 0 1 1 1
  spline S508 degree 2 poles (-19.744, -2.7348) (-19.6898, -2.7012) (-19.664, -2.6396) knots 0 0 0 1 1 1
  spline S509 degree 2 poles (-19.664, -2.6396) (-19.6382, -2.5779) (-19.6538, -2.4727) knots 0 0 0 1 1 1
  spline S510 degree 2 poles (-19.6538, -2.4727) (-19.6655, -2.3937) (-19.7031, -2.2675) knots 0 0 0 1 1 1
  line L223 (-20.304, -1.5499) -> (-22.356, -1.8388)
  line L224 (-22.356, -1.8388) -> (-23.2185, -1.8986)
  line L225 (-23.2185, -1.8986) -> (-23.2595, -1.3068)
  line L226 (-23.2595, -1.3068) -> (-22.397, -1.247)
  line L227 (-22.397, -1.247) -> (-20.3253, -1.2421)
  line L228 (-20.3253, -1.2421) -> (-20.304, -1.5499)
  line L229 (-19.3293, -1.6077) -> (-19.8734, -1.6454)
  line L230 (-19.8734, -1.6454) -> (-19.9115, -1.096)
  line L231 (-19.9115, -1.096) -> (-19.3674, -1.0583)
  line L232 (-19.3674, -1.0583) -> (-19.3293, -1.6077)
  dimension "d27" = 1.7314
extrude "Extrusion8" add sketch "Skizze8" along normal blind 0.6 contours L229 L230 L231 L232 | L64 L65 L66 S183 S184 S185 L67 S186 S187 S188 S189 L68 L69 | L75 L76 L77 L78 L79 S224 S225 S226 S227 L80 S228 S229 S230 L81 L82 L83 L84 L85 L86 | L183 L184 L185 L186 L187 S413 S414 S415 S416 L188 S417 S418 S419 L189 L190 L191 L192 L193 L194 | L0 L1 L2 S0 S1 L3 L4 L5 L6 | A2 L36 L37 L38 L39 | A2 L41 L42 L43 S84 S85 L44 L45 L46 | A2 L40 S79 S80 S81 S82 S83 L41 L46 S86 S87 S88 S89 | A2 S52 S53 S54 S55 S56 S57 S58 S59 S60 | A2 S90 S91 S92 S93 S94 S95 S96 S97 S98 | A2 L23 S35 S36 S37 S38 S39 S40 S41 S42 S43 L24 L25 L26 L27 | A2 L55 L56 L57 L58 S117 S118 S119 S120 S121 S122 S123 S124 L59 | A2 L19 L20 L21 L22 | A2 S133 S134 S135 S136 S137 S138 S139 S140 S141 | A2 L11 L12 L13 L14 | A2 S150 S151 S152 S153 S154 S155 S156 S157 S158 S159 S160 S161 S162 S163 L60 S164 S165 S166 S167 S168 S169 S170 L61 S171 S172 L62 S173 | A2 S2 S3 S4 S5 S6 S7 S8 S9 S10 S11 S12 S13 S14 S15 L7 S16 S17 S18 S19 S20 S21 S22 L8 S23 S24 L9 S25 | A2 L70 S190 S191 S192 S193 S194 S195 S196 S197 S198 L71 L72 L73 L74 | A2 L211 S503 S504 S505 S506 L212 L213 L214 L215 L216 L217 L218 L219 L220 L221 L222 S507 S508 S509 S510 | A2 S207 S208 S209 S210 S211 S212 S213 S214 S215 | A2 S470 S471 S472 S473 S474 S475 S476 S477 S478 S479 S480 S481 S482 S483 L207 S484 S485 S486 S487 S488 S489 S490 L208 S491 S492 L209 S493 | A2 L87 S231 S232 S233 S234 L88 L89 L90 L91 L92 L93 L94 L95 L96 L97 L98 S235 S236 S237 S238 | A2 S453 S454 S455 S456 S457 S458 S459 S460 S461 | A2 L107 S248 S249 S250 S251 S252 S253 S254 S255 S256 L108 S257 S258 S259 S260 | A2 L202 L203 L204 L205 S437 S438 S439 S440 S441 S442 S443 S444 L206 | A2 L199 S420 S421 S422 S423 S424 S425 S426 S427 S428 L200 S429 S430 S431 S432 | A2 L110 L111 L112 S265 S266 L113 L114 L115 L116 L117 L118 L119 L120 L121 L122 | A2 L195 L196 L197 L198 | A2 L123 S267 S268 S269 S270 S271 S272 S273 S274 S275 S276 S277 S278 S279 S280 S281 S282 S283 S284 L124 S285 S286 S287 S288 S289 S290 S291 S292 S293 S294 S295 S296 S297 S298 S299 | A2 L125 L126 L127 S300 S301 L128 L129 L130 L131 L132 L133 L134 L135 L136 L137 | A2 S396 S397 S398 S399 S400 S401 S402 S403 S404 | A2 L139 L140 L141 S307 S308 L142 L143 L144 | A2 L138 S302 S303 S304 S305 S306 L139 L144 S309 S310 S311 S312 | A2 L180 S379 S380 S381 S382 S383 S384 S385 S386 S387 L181 S388 S389 S390 S391 | A2 L145 S313 S314 S315 S316 S317 S318 S319 S320 S321 S322 S323 S324 S325 S326 S327 S328 L146 S329 S330 S331 S332 S333 S334 S335 S336 S337 S338 S339 S340 S341 S342 S343 | A2 L172 S368 S369 S370 S371 S372 L173 L174 L175 S373 S374 S375 S376 S377 S378 L176 L177 L178 L179 | A2 L147 S344 S345 S346 S347 L148 L149 L150 L151 L152 L153 L154 L155 L156 L157 L158 S348 S349 S350 S351 | A2 L167 L170 L171 | A2 L167 S352 S353 S354 S355 S356 S357 S358 S359 L168 L169 L170 | A2 L163 L164 L165 L166 | L15 L16 L17 L18 | L28 L29 L30 S69 S70 S71 S72 S73 L31 L32 L33 S74 S75 S76 S77 S78 L34 L35 | L47 L48 L49 S107 S108 S109 S110 S111 L50 L51 L52 S112 S113 S114 S115 S116 L53 L54 | L99 L100 L101 S239 S240 S241 S242 L102 L103 L104 S243 S244 S245 S246 S247 L105 L106 | L159 L160 L161 L162 | L223 L224 L225 L226 L227 L228
